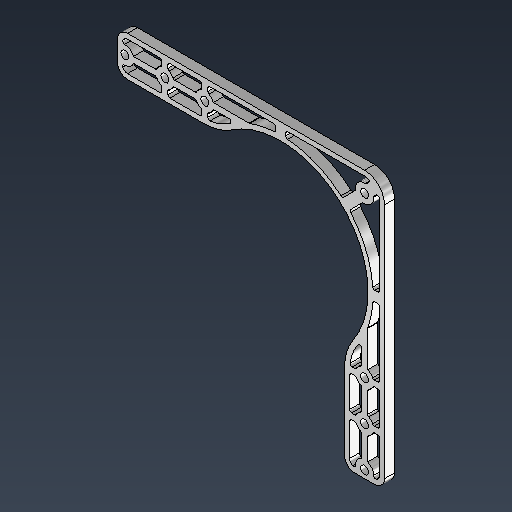
# Autodesk Inventor part: PLATE,CLAMP,MK4i,Swerve,CUSTOM
Saved by Autodesk Inventor 2026 (Build 300175050, 175E)
## iProperties
Created: 2021-12-05
Part Number: PLATE,CLAMP,MK4i,Swerve,CUSTOM
Material: Aluminum 7075
Document SubType Name: Modeling
Designer: dave.simone
Density: 2.81 g/cm^3
Appearance: Aluminum - Polished
Mass: 58.334 g
Surface Area: 175.902 cm^2
Volume: 20.7594 cm^3
Author: dave.simone
Revision Number: ANY
Autodesk Inventor part; units mm, degrees
ref_plane "Work Plane2" through (0, 0, 0) normal (-0.7071, 0.7071, 0) x (0, 0, 1)
ref_plane "XY Plane" through (0, 0, 0) normal (0, 0, 1) x (1, 0, 0)
ref_plane "Work Plane2" through (0, 0, 0) normal (-0.7071, 0.7071, 0) x (0, 0, 1)
sketch "Sketch1" plane through (-160.3375, 44.45, 0) normal (0, 0, 1) x (1, 0, 0)
  line L0 (311.15, -57.15) -> (160.3375, -57.15)
  arc A0 (311.15, -57.15) -> (317.5, -50.8) centre (311.15, -50.8) ccw
  line L1 (317.5, -38.1) -> (317.5, -50.8)
  arc A1 (317.5, -38.1) -> (311.15, -31.75) centre (311.15, -38.1) ccw
  line L2 (262.4883, -31.75) -> (311.15, -31.75)
  arc A2 (262.4883, -31.75) -> (244.7389, -37.1747) centre (262.4883, -63.5) ccw
  arc A3 (167.6111, 39.9604) -> (244.7389, -37.1747) centre (213.6775, 8.8946) ccw
  arc A4 (167.6111, 39.9604) -> (173.0375, 57.7122) centre (141.2875, 57.7122) ccw
  line L3 (173.0375, 106.3625) -> (173.0375, 57.7122)
  arc A5 (173.0375, 106.3625) -> (166.6875, 112.7125) centre (166.6875, 106.3625) ccw
  line L4 (153.9875, 112.7125) -> (166.6875, 112.7125)
  arc A6 (153.9875, 112.7125) -> (147.6375, 106.3625) centre (153.9875, 106.3625) ccw
  line L5 (147.6375, -44.45) -> (147.6375, 106.3625)
  arc A7 (147.6375, -44.45) -> (160.3375, -57.15) centre (160.3375, -44.45) ccw
  line L6 (160.3375, -105.5571) -> (160.3375, 150.6251) construction
  line L7 (99.2247, -44.45) -> (355.4135, -44.45) construction
  dimension "d0" = 55.5625
  dimension "d1" = 169.8625
  dimension "d2" = 12.7
  dimension "d3" = 66.0446
  dimension "d4" = 66.04
  dimension "d5" = 25.4
  dimension "d6" = 25.4
  dimension "d7" = 31.75
  dimension "d8" = 6.35
  constraints: 16 point on circle, 14 tangent, 12 end point, 8 centre point, 4 equal radius, 3 perpendicular, 2 parallel, 1 horizontal
  measures "d0" radius of A3
  measures "d1" distance between parallel lines of L1 L5
  measures "d2" radius of A7
  measures "d3" distance from line of A3.centre L0
  measures "d4" distance from line of L5 A3.centre
  measures "d5" distance between parallel lines of L2 L0
  measures "d6" distance between parallel lines of L5 L3
  measures "d7" radius of A2
  measures "d8" radius of A0
extrude "Extrusion1" add sketch "Sketch1" along normal mid plane 6.35
sketch "Sketch2" plane through (-160.3375, 44.45, 3.175) normal (0, 0, 1) x (1, 0, 0)
  line L0 (160.3375, -91.1225) -> (160.3375, 146.685) construction
  line L1 (113.665, -44.45) -> (351.4725, -44.45) construction
  line L2 (317.5, -50.8) -> (317.5, -38.1) construction
  point P0 (160.3375, -44.45)
  point P1 (312.7375, -44.45)
  dimension "d13" = 152.4
  constraints: 1 point on line
  measures "d13" distance from line of L0 point (312.738, -44.45)
hole "Hole1" at (152.4, 0, 3.175) direction (0, 0, -1) diameter 5.1054 end through all clearance for "Socket Head Cap Screw" size "#10" standard "Ansi Unified Screw Threads"
pattern_linear "Rectangular Pattern1" count 3 spacing 25.4 along (-1, 0, 0) of "Hole1"
sketch "Sketch4" plane through (-160.3375, 44.45, 3.175) normal (0, 0, 1) x (1, 0, 0)
  point P0 (160.3375, -44.45)
  point P1 (160.3375, -44.45)
  constraints: 1 coincident
hole "Hole2" at (0, 0, 3.175) direction (0, 0, -1) diameter 5.1054 end through all clearance for "Socket Head Cap Screw" size "#10" standard "Ansi Unified Screw Threads"
sketch "Sketch3" plane through (-160.3375, 44.45, 3.175) normal (0, 0, 1) x (1, 0, 0)
  circle A0 centre (261.9375, -44.45) radius 2.5527 projected
  circle A1 centre (287.3375, -44.45) radius 2.5527 projected
  circle A2 centre (312.7375, -44.45) radius 2.5527 projected
  line L0 (311.15, -31.75) -> (262.4883, -31.75) projected
  arc A3 (262.4883, -31.75) -> (244.7389, -37.1747) centre (262.4883, -63.5) ccw projected
  arc A4 (167.6111, 39.9604) -> (244.7389, -37.1747) centre (213.6775, 8.8946) ccw projected
  arc A5 (167.6111, 39.9604) -> (173.0375, 57.7122) centre (141.2875, 57.7122) ccw construction
  line L1 (173.0375, 57.7122) -> (173.0375, 106.3625) construction
  arc A6 (173.0375, 106.3625) -> (166.6875, 112.7125) centre (166.6875, 106.3625) ccw construction
  line L2 (166.6875, 112.7125) -> (153.9875, 112.7125) construction
  arc A7 (153.9875, 112.7125) -> (147.6375, 106.3625) centre (153.9875, 106.3625) ccw construction
  line L3 (147.6375, 106.3625) -> (147.6375, -44.45) construction
  arc A8 (147.6375, -44.45) -> (160.3375, -57.15) centre (160.3375, -44.45) ccw projected
  line L4 (160.3375, -57.15) -> (311.15, -57.15) projected
  arc A9 (311.15, -57.15) -> (317.5, -50.8) centre (311.15, -50.8) ccw projected
  line L5 (317.5, -50.8) -> (317.5, -38.1) projected
  arc A10 (317.5, -38.1) -> (311.15, -31.75) centre (311.15, -38.1) ccw projected
  circle A11 centre (312.7375, -44.45) radius 5.7277
  circle A12 centre (287.3375, -44.45) radius 5.7277
  circle A13 centre (261.9375, -44.45) radius 5.7277
  line L6 (151.3572, -53.4303) -> (174.387, -30.3922) construction
  arc A14 (311.15, -53.975) -> (314.325, -50.8) centre (311.15, -50.8) ccw
  line L7 (311.15, -53.975) -> (160.3375, -53.975)
  arc A15 (150.8125, -44.45) -> (160.3375, -53.975) centre (160.3375, -44.45) ccw
  line L8 (150.8125, -44.45) -> (150.8125, 106.3625)
  arc A16 (153.9875, 109.5375) -> (150.8125, 106.3625) centre (153.9875, 106.3625) ccw
  line L9 (153.9875, 109.5375) -> (166.6875, 109.5375)
  arc A17 (169.8625, 106.3625) -> (166.6875, 109.5375) centre (166.6875, 106.3625) ccw
  line L10 (169.8625, 106.3625) -> (169.8625, 57.7122)
  arc A18 (164.9788, 41.7356) -> (169.8625, 57.7122) centre (141.2875, 57.7122) ccw
  arc A19 (164.9788, 41.7356) -> (246.5138, -39.8072) centre (213.6775, 8.8946) ccw
  arc A20 (262.4883, -34.925) -> (246.5138, -39.8072) centre (262.4883, -63.5) ccw
  line L11 (262.4883, -34.925) -> (311.15, -34.925)
  arc A21 (314.325, -38.1) -> (311.15, -34.925) centre (311.15, -38.1) ccw
  line L12 (314.325, -38.1) -> (314.325, -50.8)
  line L13 (307.3359, -46.355) -> (292.7391, -46.355)
  line L14 (281.9359, -46.355) -> (267.3391, -46.355)
  line L15 (256.5359, -46.355) -> (233.6168, -46.355)
  line L16 (307.3359, -42.545) -> (292.7391, -42.545)
  line L17 (281.9359, -42.545) -> (267.3391, -42.545)
  line L18 (256.5359, -42.545) -> (242.0335, -42.545)
  line L19 (289.2425, -53.975) -> (289.2425, -49.8516)
  line L20 (285.4325, -53.975) -> (285.4325, -49.8516)
  line L21 (289.2425, -39.0484) -> (289.2425, -34.925)
  line L22 (285.4325, -39.0484) -> (285.4325, -34.925)
  line L23 (263.8425, -53.975) -> (263.8425, -49.8516)
  line L24 (260.0325, -53.975) -> (260.0325, -49.8516)
  line L25 (263.8425, -39.0484) -> (263.8425, -34.925)
  line L26 (260.0325, -39.0484) -> (260.0325, -35.0307)
  line L27 (174.4481, -34.822) -> (156.2319, -53.0448)
  line L28 (216.8525, -53.975) -> (216.8525, -49.757)
  line L29 (210.5025, -53.975) -> (210.5025, -49.757)
  circle A22 centre (160.3375, -44.45) radius 2.5527 construction
  circle A23 centre (160.3375, -44.45) radius 5.7277
  point P0 (314.325, -49.9533)
  point P1 (314.325, -38.9467)
  point P2 (165.9527, -43.3204)
  point P3 (159.21, -50.0656)
  dimension "d25" = 3.175
  dimension "d26" = 3.175
  dimension "d27" = 3.81
  dimension "d28" = 3.81
  dimension "d29" = 3.81
  dimension "d30" = 6.35
  dimension "d31" = 3.175
  constraints: 48 end point, 27 point on circle, 21 point on line, 10 centre point, 8 parallel, 4 vertical, 2 collinear, 1 horizontal, 1 perpendicular, 35 other
  measures "d25" distance between parallel lines of L4 L7
  measures "d26" radial gap between concentric circles of A11 A2
  measures "d27" distance between parallel lines of L13 L16
  measures "d28" distance between parallel lines of L20 L19
  measures "d29" distance between parallel lines of L24 L23
  measures "d30" distance between parallel lines of L29 L28
  measures "d31" distance between parallel lines of L27 L6
extrude "Extrusion2" cut sketch "Sketch3" against normal through all contours A11 L16 A12 L21 L11 A21 L12 | L12 A14 L7 L19 A12 L13 A11 | A12 L17 A13 L25 L11 L22 | L20 L7 L23 A13 L14 A12 | L7 L28 A19 L15 A13 L24 | L26 A13 L18 A19 A20 | L7 A15 L27 A23 A19 L29
fillet "Fillet1" radius 1.27 35 edges at (153.9875, -5.5033, 0) (153.9875, 5.5033, 0) (128.905, -9.525, 0) (128.905, -5.4016, 0) (132.4016, -1.905, 0) (132.4016, 1.905, 0) (128.905, 5.4016, 0) (128.905, 9.525, 0) (125.095, 5.4016, 0) (125.095, 9.525, 0) (121.5984, 1.905, 0) (107.0016, 1.905, 0) (103.505, 5.4016, 0) (103.505, 9.525, 0) (125.095, -9.525, 0) (125.095, -5.4016, 0) (121.5984, -1.905, 0) (107.0016, -1.905, 0) (103.505, -5.4016, 0) (103.505, -9.525, 0) (99.695, -9.525, 0) (99.695, -5.4016, 0) (96.1984, 1.905, 0) (99.695, 5.4016, 0) (99.695, 9.4193, 0) (81.696, 1.905, 0) (56.515, -5.307, 0) (56.515, -9.525, 0) (50.165, -9.525, 0) (50.165, -5.307, 0) (14.1106, 9.628, 0) (-4.1056, -8.5948, 0) (73.2793, -1.905, 0) (-1.1275, -5.6156, 0) (5.6152, 1.1296, 0)
mirror "Mirror1" about plane through (0, 0, 0) normal (-0.7071, 0.7071, 0) of "Extrusion2", "Fillet1", "Hole1", "Rectangular Pattern1"
equation "\"d28\" = d27"
equation "\"d29\" = d28"
body "Solid18"
